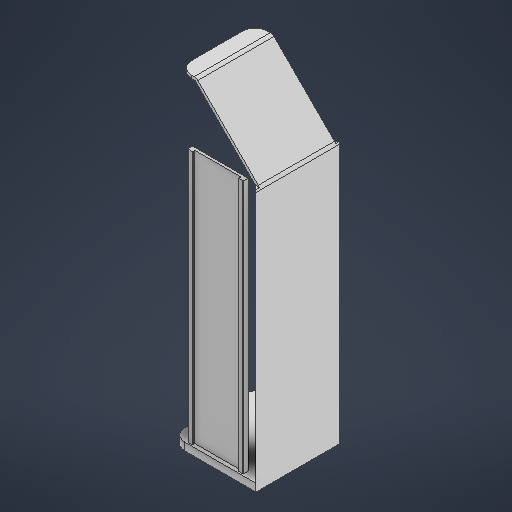
# Autodesk Inventor part: bottom_frame
Saved by Autodesk Inventor 2027 (Build 310192060, 192F)
## iProperties
Created: 2026-07-05
Part Number: bottom_frame
Material: Ogólny
Document SubType Name: Modeling
Designer: User
Density: 1 g/cm^3
Appearance: Domyślna
Author: User
Autodesk Inventor part; units mm, degrees
ref_plane "YZ Plane" through (0, 0, 0) normal (1, 0, 0) x (0, 1, 0)
ref_plane "XZ Plane" through (0, 0, 0) normal (0, 1, 0) x (-1, 0, 0)
ref_plane "XY Plane" through (0, 0, 0) normal (0, 0, 1) x (1, 0, 0)
sketch "Szkic1" plane through (0, 0, 0) normal (0, 1, 0) x (-1, 0, 0)
  line L0 (-16.5, -16.5) -> (16.5, -16.5)
  line L1 (16.5, -16.5) -> (16.5, 16.5)
  line L2 (16.5, 16.5) -> (-16.5, 16.5)
  line L3 (-16.5, 16.5) -> (-16.5, -16.5)
  line L4 (-16.5, -16.5) -> (16.5, 16.5) construction
  line L5 (16.5, -16.5) -> (-16.5, 16.5) construction
  line L6 (-16, -16) -> (16, -16)
  line L7 (16, -16) -> (16, 16)
  line L8 (16, 16) -> (-16, 16)
  line L9 (-16, 16) -> (-16, -16)
  line L10 (-16, -16) -> (16, 16) construction
  line L11 (16, -16) -> (-16, 16) construction
  line L12 (-16, 16) -> (-16.5, 16.5)
  line L13 (-16, -16) -> (-16.5, -16.5)
  point P0 (0, 0)
  dimension "d0" = 33
  dimension "d1" = 33
  dimension "d2" = 32
  dimension "d3" = 32
  constraints: 28 end point, 4 midpoint, 4 parallel, 2 horizontal, 2 perpendicular
  measures "d0" distance of L2.end L1.end
  measures "d1" distance of L1.end L0.end
  measures "d2" distance of L8.end L7.end
  measures "d3" distance of L7.end L6.end
extrude "Wyciągnięcie proste1" add sketch "Szkic1" against normal blind 3
sketch "Szkic2" plane through (0, 0, 0) normal (0, 1, 0) x (1, 0, 0)
  line L0 (15, 15) -> (-15, 15)
  line L1 (-15, 15) -> (-15, -15)
  line L2 (-15, -15) -> (15, -15)
  line L3 (15, -15) -> (15, 15)
  line L4 (15, 15) -> (-15, -15) construction
  line L5 (-15, 15) -> (15, -15) construction
  line L6 (-15, -15) -> (-11, -15)
  line L7 (-11, -15) -> (-11, -15.9)
  line L8 (-11, -15.9) -> (-9.1, -15.9)
  line L9 (-9.1, -15.9) -> (-9.1, -15)
  line L10 (-9.1, -15.9) -> (-8.2, -15.9) construction
  line L11 (9, -15) -> (9, -15.9)
  line L12 (9, -15.9) -> (10.9, -15.9)
  line L13 (10.9, -15.9) -> (10.9, -15)
  line L14 (10.9, -15.9) -> (11.8, -15.9) construction
  line L15 (-15, 0) -> (15, 0) construction
  line L16 (-11, 15) -> (-11, 15.9)
  line L17 (-11, 15.9) -> (-9.1, 15.9)
  line L18 (-9.1, 15.9) -> (-9.1, 15)
  line L19 (-9.1, 15.9) -> (-8.2, 15.9) construction
  line L20 (9, 15) -> (9, 15.9)
  line L21 (9, 15.9) -> (10.9, 15.9)
  line L22 (10.9, 15.9) -> (10.9, 15)
  line L23 (10.9, 15.9) -> (11.8, 15.9) construction
  line L24 (-11, -15) -> (10.9, -15)
  line L25 (10.9, -15) -> (10.9, -14)
  line L26 (10.9, -14) -> (-11, -14)
  line L27 (-11, -14) -> (-11, -15)
  line L28 (-11, 15) -> (10.9, 15)
  line L29 (10.9, 15) -> (10.9, 14)
  line L30 (10.9, 14) -> (-11, 14)
  line L31 (-11, 14) -> (-11, 15)
  point P0 (0, 0)
  dimension "d6" = 30
  dimension "d7" = 30
  dimension "d8" = 4
  dimension "d9" = 0.9
  dimension "d10" = 1.9
  dimension "d12" = 0.9
  dimension "d13" = 90
  dimension "d16" = 20
  dimension "d23" = 21.9
  dimension "d24" = 1
  dimension "d25" = 1
  constraints: 64 end point, 10 symmetric about line, 7 perpendicular, 6 parallel, 4 midpoint, 3 horizontal, 1 point on line, 9 other
  measures "d6" distance of L2.end L1.end
  measures "d7" distance of L1.end L0.end
  measures "d8" distance of L1.end L6.end
  measures "d9" distance of L6.end L7.end
  measures "d10" distance of L7.end L8.end
  measures "d12" distance of L8.end L9.end
  measures "d13" angle of L10 L9
  measures "d16" distance of L7.end L11.end
  measures "d23" distance of L6.end L13.end
  measures "d24" distance of L25.end L13.end
  measures "d25" distance of L22.end L29.end
extrude "Wyciągnięcie proste2" add sketch "Szkic2" along normal blind 100 contours L29 L30 L31 L0 | L0 L20 L21 L22 | L13 L12 L11 L2 | L2 L27 L26 L25 | L0 L16 L17 L18 | L9 L8 L7 L2
fillet "Zaokrąglenie1" radius 0.2 8 edges at (-9.1, 50, 15.9) (-11, 50, 15.9) (10.9, 50, 15.9) (9, 50, 15.9) (10.9, 50, -15.9) (9, 50, -15.9) (-9.1, 50, -15.9) (-11, 50, -15.9)
sketch "Szkic3" plane through (0, 0, 0) normal (0, 1, 0) x (1, 0, 0)
  line L0 (15, -15) -> (-15, -15)
  line L1 (-15, -15) -> (-15, 15)
  line L2 (-15, 15) -> (15, 15)
  line L3 (15, 15) -> (15, -15)
  line L4 (15, -15) -> (-15, 15) construction
  line L5 (-15, -15) -> (15, 15) construction
  line L6 (16.5, -16.5) -> (16.5, 16.5) projected
  line L7 (15, -15) -> (16.5, -16.5)
  line L8 (15, 15) -> (16.5, 16.5)
  line L9 (-16.5, -16.5) -> (16.5, -16.5)
  line L10 (16.5, -16.5) -> (16.5, 16.5)
  line L11 (16.5, 16.5) -> (-16.5, 16.5)
  line L12 (-16.5, 16.5) -> (-16.5, -16.5)
  line L13 (-16.5, -16.5) -> (16.5, 16.5) construction
  line L14 (16.5, -16.5) -> (-16.5, 16.5) construction
  line L15 (-16.5, 16.5) -> (16.5, 16.5)
  line L16 (16.5, 16.5) -> (16.5, -16.5)
  line L17 (16.5, -16.5) -> (-16.5, -16.5)
  line L18 (-16.5, -16.5) -> (-16.5, 16.5)
  line L19 (-16.5, 16.5) -> (16.5, -16.5) construction
  line L20 (16.5, 16.5) -> (-16.5, -16.5) construction
  point P0 (0, 0)
  dimension "d27" = 30
  dimension "d28" = 30
  constraints: 40 end point, 6 midpoint, 6 parallel, 3 horizontal, 3 perpendicular
  measures "d27" distance of L1.end L2.end
  measures "d28" distance of L0.end L1.end
extrude "Wyciągnięcie proste3" add sketch "Szkic3" along normal blind 100 contours L3 L8 L6 L7
fillet "Zaokrąglenie2" radius 5 2 edges at (-16.5, -1.5, 16.5) (-16.5, -1.5, -16.5)
ref_plane "Płaszczyzna konstrukcyjna1" through (16.5, 100, 16.5) normal (0.7071068, 0.7071068, 0) x (0, 0, -1)
sketch "Szkic4" plane through (16.5, 100, 16.5) normal (0.7071068, 0.7071068, 0) x (0, 0, -1)
  line L0 (31.5, 1.0607) -> (1.5, 1.0607) projected
  line L1 (16.5, 1.0607) -> (16.5, 17.8607)
  line L2 (16.5, 1.0607) -> (33.3, 1.0607) construction
  line L3 (1.5, 0.3607) -> (31.5, 0.3607)
  line L4 (31.5, 0.3607) -> (31.5, 35.3607)
  line L5 (31.5, 35.3607) -> (1.5, 35.3607)
  line L6 (1.5, 35.3607) -> (1.5, 0.3607)
  line L7 (1.5, 0.3607) -> (31.5, 35.3607) construction
  line L8 (31.5, 0.3607) -> (1.5, 35.3607) construction
  point P0 (16.5, -59.0434)
  point P1 (1.5, 1.0607)
  dimension "d34" = 16.8
  dimension "d35" = 90
  dimension "d36" = 30
  dimension "d37" = 35
  constraints: 16 end point, 3 midpoint, 2 horizontal, 2 parallel, 2 perpendicular, 1 vertical
  measures "d34" distance of L1.start L1.end
  measures "d35" angle of L2 L1
  measures "d36" distance of L5.end L4.end
  measures "d37" distance of L4.end L3.end
extrude "Wyciągnięcie proste4" add sketch "Szkic4" against normal blind 1.2 contours L0 L6 L5 L4
ref_plane "Płaszczyzna konstrukcyjna2" through (-8.5038, 125.0038, -15) normal (0, 1, 0) x (0, 0, 1)
sketch "Szkic5" plane through (-8.5038, 125.0038, -15) normal (0, 1, 0) x (0, 0, 1)
  line L0 (30, -0.8485) -> (0, -0.8485) projected
  line L1 (15, -0.8485) -> (15, -3.8485)
  line L2 (0, -6.8485) -> (30, -6.8485)
  line L3 (30, -6.8485) -> (30, -0.8485)
  line L4 (30, -0.8485) -> (0, -0.8485)
  line L5 (0, -0.8485) -> (0, -6.8485)
  line L6 (0, -6.8485) -> (30, -0.8485) construction
  line L7 (30, -6.8485) -> (0, -0.8485) construction
  point P0 (15, 8.5038)
  dimension "d41" = 3
  dimension "d42" = 30
  dimension "d43" = 6
  constraints: 14 end point, 3 midpoint, 2 parallel, 1 horizontal, 1 perpendicular, 1 vertical
  measures "d41" distance of L1.start L1.end
  measures "d42" distance of L4.end L3.end
  measures "d43" distance of L3.end L2.end
extrude "Wyciągnięcie proste5" add sketch "Szkic5" against normal blind 1.2
fillet "Zaokrąglenie4" radius 5 2 edges at (-15.3523, 124.4038, 15) (-15.3523, 124.4038, -15)
sketch "Szkic6" plane through (15.75, 100.75, 15) normal (0, 0, 1) x (0.7071068, 0.7071068, 0)
  line L0 (-1.2, 34.3) -> (-1.4485, 34.0515) projected
  line L1 (-0.6, 34.9) -> (-1.3071, 35.6071) projected
  line L2 (-1.2, 34.3) -> (-0.6, 34.9)
  line L3 (0, 34.3) -> (0, 0) projected
  line L4 (-0.6, 34.9) -> (0, 34.3)
  line L5 (-1.2, 34.3) -> (-1.2, 0) projected
  line L6 (0, 34.3) -> (-1.2, 34.3)
  line L7 (-2.1556, 34.7586) -> (-1.4485, 34.0515) projected
  line L8 (-1.2, 34.3) -> (-1.4485, 34.0515)
  line L9 (-1.4485, 34.0515) -> (-1.2, 33.8029)
  line L10 (-1.2, 33.8029) -> (-1.2, 34.3)
  line L11 (-1.2, 0) -> (-1.2, -0.1393)
  line L12 (-71.7713, -70.7107) -> (-1.0607, 0) projected
  line L13 (0, -1.0607) -> (-1.0607, 0) projected
  line L14 (-1.0607, 0) -> (-1.2, -0.1393)
  line L15 (-1.0607, 0) -> (0, -1.0607)
  line L16 (0, -1.0607) -> (0, 0)
  line L17 (0, 0) -> (-1.0607, 0) projected
  line L18 (0, 0) -> (-1.0607, 0)
  line L19 (-1.0607, 0) -> (-1.2, 0)
  point P0 (-82.3779, -60.1041)
  constraints: 24 end point, 5 perpendicular, 4 collinear, 1 parallel, 1 point on line, 1 vertical
extrude "Wyciągnięcie proste6" add sketch "Szkic6" against normal up to surface (30 mm away)
fillet "Zaokrąglenie5" radius 2 2 edges at (-8.5038, 125.0038, 0) (16.5, 100, 0)
